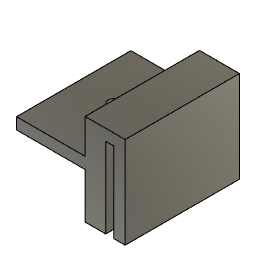
Limit_Interrupter v4 (Autodesk Fusion 360 design; units mm, degrees)
Autodesk Fusion 360 part; units mm, degrees
sketch "Sketch1" plane through (0, 0, 0) normal (0, 1, 0) x (1, 0, 0) in component "Limit Interrupter"
  line L0 (0, 0) -> (0, -7.014)
  line L1 (0, -7.014) -> (1.5, -7.014)
  line L2 (1.5, -7.014) -> (1.5, 0)
  line L3 (1.5, 0) -> (2.5, 0)
  line L4 (2.5, 0) -> (2.5, -8)
  line L5 (2.5, -8) -> (-1, -8)
  line L6 (-1, -8) -> (-1, 0)
  line L7 (-1, 0) -> (0, 0)
  line L8 (-1, -4.9804) -> (-7, -4.9804)
  line L9 (-7, -4.9804) -> (-7, -3.9804)
  line L10 (-7, -3.9804) -> (-1, -3.9804)
  dimension "d1" = 1
  dimension "d2" = 3.5
  dimension "d3" = 1.5
  dimension "d4" = 6
  dimension "d5" = 1
  dimension "d6" = 8
  dimension "d7" = 8
  constraint coincident L0.start L7.end
  constraint vertical L0
  constraint perpendicular L0 L1
  constraint perpendicular L1 L2
  constraint perpendicular L2 L3
  constraint perpendicular L3 L4
  constraint perpendicular L4 L5
  constraint perpendicular L5 L6
  constraint perpendicular L0 L7
  constraint coincident L6 L8.start
  constraint perpendicular L6 L8
  constraint perpendicular L8 L9
  constraint coincident L6 L10.end
  constraint perpendicular L6 L10
  measures "d1" distance of L2.end L3.end
  measures "d2" distance of L4.end L5.end
  measures "d3" distance of L0.end L1.end
  measures "d4" distance of L8.start L8.end
  measures "d5" distance of L8.end L9.end
  measures "d6" distance of L3.end L4.end
  measures "d7" distance of L5.end L6.end
extrude "Extrude1" add sketch "Sketch1" along normal blind 10 in component "Limit Interrupter"
hole "Hole1" at (-3.7627, 5.2663, 4.9804) direction (0, 0, -1) diameter 1 depth 2 tip angle 118 in component "Limit Interrupter"
sketch "Sketch1 (2)" plane through (0, 0, 0) normal (0, -1, 0) x (1, 0, 0)
  line L0 (-7, 4.9804) -> (-7, 3.9804)
  line L1 (-7, 3.9804) -> (-1, 3.9804)
  line L2 (-1, 3.9804) -> (-1, 0)
  line L3 (-1, 0) -> (0, 0)
  line L4 (0, 0) -> (0, 7.014)
  line L5 (0, 7.014) -> (1.5, 7.014)
  line L6 (1.5, 7.014) -> (1.5, 0)
  line L7 (1.5, 0) -> (2.5, 0)
  line L8 (2.5, 0) -> (2.5, 8)
  line L9 (2.5, 8) -> (-1, 8)
  line L10 (-1, 8) -> (-1, 4.9804)
  line L11 (-1, 4.9804) -> (-7, 4.9804)
  line L12 (0, 0) -> (0.8, 0)
  line L13 (0.8, 0) -> (0.8, 7.014)
  line L14 (0.8, 7.014) -> (0, 7.014)
  dimension "d13" = 0.8
  dimension "d14" = 7.014
  constraint coincident L3.end L4.start
  constraint perpendicular L4 L12
  constraint perpendicular L12 L13
  constraint coincident L4 L5.start
  constraint perpendicular L4 L14
  measures "d13" distance of L3.end L12.end
  measures "d14" distance of L12.end L13.end
extrude "Extrude2" add sketch "Sketch1 (2)" against normal blind 0.8 contours L4 L5 L12 L13 L14 in component "Limit Interrupter"
component "Limit Interrupter" placed x (1, 0, 0) y (0, 1, 0) z (0, 0, 1) at (0, 0, 0)
